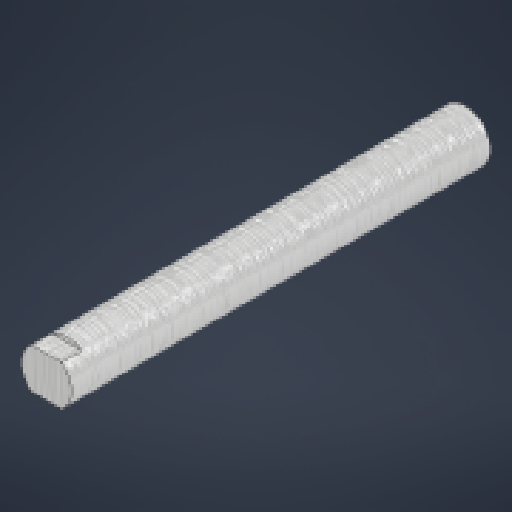
# Autodesk Inventor part: shaft_tibea
Saved by Autodesk Inventor 2026 (Build 300175000, 175)
## iProperties
Created: 2026-04-24
Part Number: shaft_tibea
Material: Сталь 09Г2С
Document SubType Name: Modeling
Designer: user
Density: 7.85 g/cm^3
Appearance: Полированный — шлифованный
Mass: 172.535 g
Surface Area: 62.3609 cm^2
Volume: 21.979 cm^3
Author: user
Autodesk Inventor part; units mm, degrees
ref_plane "YZ Plane" through (0, 0, 0) normal (1, 0, 0) x (0, 1, 0)
ref_plane "XZ Plane" through (0, 0, 0) normal (0, 1, 0) x (-1, 0, 0)
ref_plane "XY Plane" through (0, 0, 0) normal (0, 0, 1) x (1, 0, 0)
sketch "Эскиз1" plane through (0, 0, 0) normal (0, 0, 1) x (1, 0, 0)
  circle A0 centre (0, 0) radius 7.5
  dimension "d0" = 15
  constraints: 1 centre point, 1 coincident
  measures "d0" diameter of A0
extrude "Выдавливание1" add sketch "Эскиз1" along normal blind 124.5
sketch "Эскиз2" plane through (0, 0, 124.5) normal (0, 0, 1) x (1, 0, 0)
  circle A0 centre (0, 0) radius 7.5 projected
  line L0 (4.5, 6) -> (-4.5, 6)
  line L1 (-4.5, -6) -> (4.5, -6)
  dimension "d3" = 12
  constraints: 4 end point, 4 point on circle, 2 parallel, 1 horizontal
  measures "d3" distance between parallel lines of L1 L0
extrude "Выдавливание2" cut sketch "Эскиз2" against normal blind 6 contours L0 A0 | A0 L1
equation "\"d0\" = d_main_shaft"
equation "\"d3\" = width_flattened_surface"
equation "\"d_main_shaft\" = 15"
equation "\"tolerance_plazma\" = 0.1"
equation "\"thickness_steel\" = 3"
equation "\"d_main_screw_holes\" = 6.1"
equation "\"thickness_profile_tibea\" = 3"
equation "\"thickness_profile_femur\" = 3"
equation "\"width_flattened_surface\" = 12"
equation "\"width_shaft_shift\" = 35"
equation "\"hight_shaft_shift\" = 37"
